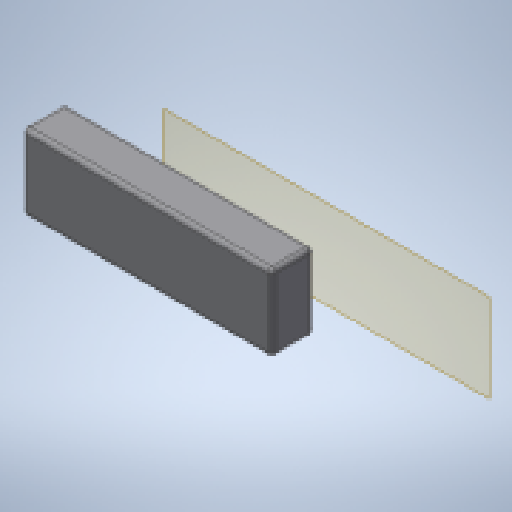
# Autodesk Inventor part: 电池
Saved by Autodesk Inventor 2025.2 (Build 292293000, 293)
## iProperties
Created: 2025-09-29
Part Number: 电池
Material: 常规
Document SubType Name: Modeling
Designer: BO‘S_SLAVE
Density: 1 g/cm^3
Appearance: 默认
Author: BO‘S_SLAVE
Autodesk Inventor part; units mm, degrees
ref_plane "YZ Plane" through (0, 0, 0) normal (1, 0, 0) x (0, 1, 0)
ref_plane "XZ Plane" through (0, 0, 0) normal (0, 1, 0) x (-1, 0, 0)
ref_plane "XY Plane" through (0, 0, 0) normal (0, 0, 1) x (1, 0, 0)
ref_plane "工作平面1" through (0, 0, 50) normal (0, 0, 1) x (1, 0, 0)
sketch "草图1" plane through (0, 0, 50) normal (0, 0, 1) x (1, 0, 0)
  line L0 (0, 0) -> (-118, 0)
  line L1 (-118, 0) -> (-118, -36)
  line L2 (-118, -36) -> (0, -36)
  line L3 (0, -36) -> (0, 0)
  dimension "d0" = 118
  dimension "d1" = 36
  constraints: 8 end point, 2 parallel, 1 horizontal, 1 perpendicular
  measures "d0" distance between parallel lines of L1 L3
  measures "d1" distance between parallel lines of L0 L2
extrude "拉伸1" add sketch "草图1" along normal blind 23
fillet "圆角1" radius 2 12 edges at (0, -36, 61.5) (-59, -36, 73) (0, -18, 73) (0, -18, 50) (0, 0, 61.5) (-59, -36, 50) (-59, 0, 50) (-59, 0, 73) (-118, -18, 50) (-118, 0, 61.5) (-118, -18, 73) (-118, -36, 61.5)
